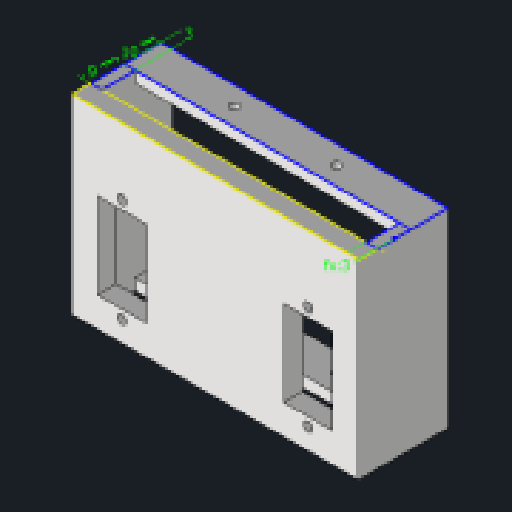
# Autodesk Inventor part: Test Frame
Saved by Autodesk Inventor 2023.2 (Build 272271030, 271C)
## iProperties
Created: 2023-10-24
Part Number: Test Frame
Material: Generic
Document SubType Name: Modeling
Designer: robpl
Density: 1 g/cm^3
Appearance: Default
Author: robpl
## iProperties of the stored document Test Frame_3DPrint.ipt
Created: 2023-10-25
Part Number: Test Frame_3DPrint
Material: Generic
Document SubType Name: Modeling
Designer: robpl
Density: 1 g/cm^3
Appearance: Default
Author: robpl
Autodesk Inventor part; units mm, degrees
ref_plane "YZ Plane" through (0, 0, 0) normal (1, 0, 0) x (0, 1, 0)
ref_plane "XZ Plane" through (0, 0, 0) normal (0, 1, 0) x (-1, 0, 0)
ref_plane "XY Plane" through (0, 0, 0) normal (0, 0, 1) x (1, 0, 0)
sketch "Sketch1" plane through (0, 0, 0) normal (0, 0, 1) x (1, 0, 0)
  line L0 (0, 0) -> (-77, 0)
  line L1 (-77, 0) -> (-77, -51.3)
  line L2 (-77, -51.3) -> (0, -51.3)
  line L3 (0, -51.3) -> (0, 0)
  line L4 (-7, -20.3) -> (-20, -20.3)
  line L5 (-20, -20.3) -> (-20, -43.3)
  line L6 (-20, -43.3) -> (-7, -43.3)
  line L7 (-7, -43.3) -> (-7, -20.3)
  line L8 (-57, -20.3) -> (-70, -20.3)
  line L9 (-70, -20.3) -> (-70, -43.3)
  line L10 (-70, -43.3) -> (-57, -43.3)
  line L11 (-57, -43.3) -> (-57, -20.3)
  point P0 (-7, -31.8)
  point P1 (0, -25.65)
  point P2 (-13.5, -20.3)
  point P3 (-63.5, -20.3)
  dimension "d1" = 51.3
  dimension "d4" = 23
  dimension "d5" = 13
  dimension "d7" = 7
  dimension "d18" = 50
  dimension "d19" = 7
  dimension "d20" = 8
  constraints: 24 end point, 6 parallel, 4 midpoint, 3 horizontal, 3 perpendicular, 2 equal length, 1 horizontal alignment
  measures "d1" distance of L1.end L0.end
  measures "d4" distance of L6.end L4.start
  measures "d5" distance of L4.start L4.end
  measures "d7" distance between parallel lines of L3 L7
  measures "d18" distance of point (-13.5, -20.3) point (-63.5, -20.3)
  measures "d19" distance between parallel lines of L1 L9
  measures "d20" distance between parallel lines of L2 L6
extrude "Extrusion1" add sketch "Sketch1" along normal blind 5
sketch "Sketch3" plane through (0, 0, 5) normal (0, 0, 1) x (1, 0, 0)
  line L0 (-77, 0) -> (-77, -51.3) projected
  line L1 (-77, -51.3) -> (0, -51.3) projected
  line L2 (0, -51.3) -> (0, 0) projected
  line L3 (0, 0) -> (-77, 0) projected
  line L4 (-7, -20.3) -> (-7, -43.3) projected
  line L5 (-7, -43.3) -> (-20, -43.3) projected
  line L6 (-20, -43.3) -> (-20, -20.3) projected
  line L7 (-20, -20.3) -> (-7, -20.3) projected
  line L8 (-20, -20.3) -> (-7, -20.3) projected
  line L9 (-70, -20.3) -> (-57, -20.3) projected
  point P0 (-13.5, -17.9)
  point P1 (-13.5, -45.7)
  point P2 (-13.5, -20.3)
  point P3 (-13.5, -20.3)
  point P4 (-13.5, -43.3)
  point P5 (-63.5, -17.9)
  point P6 (-63.5, -45.7)
  point P7 (-63.5, -20.3)
  point P8 (-63.5, -20.3)
  dimension "d8" = 27.8
  dimension "d9" = 2.4
  dimension "d10" = 2.4
  constraints: 5 midpoint, 4 vertical alignment, 2 horizontal alignment
  measures "d8" distance of point (-13.5, -17.9) point (-13.5, -45.7)
  measures "d9" distance from line of L7 point (-13.5, -17.9)
  measures "d10" distance of point (-13.5, -45.7) point (-13.5, -43.3)
hole "Hole1" at (-13.5, -17.9, 5) at (-13.5, -45.7, 5) at (-63.5, -45.7, 5) at (-63.5, -17.9, 5) direction (0, 0, -1) diameter 2.5 end through all
sketch "Sketch4" plane through (-77, 0, 0) normal (0, 1, 0) x (1, 0, 0)
  line L0 (77, 0) -> (0, 0) projected
  line L1 (0, 0) -> (0, -5) projected
  line L2 (77, -5) -> (0, -5) projected
  line L3 (77, 0) -> (77, -5) projected
  line L4 (77, 20) -> (0, 20)
  line L5 (0, 20) -> (0, 8)
  line L6 (0, 8) -> (77, 8)
  line L7 (77, 8) -> (77, 20)
  line L8 (0, 0) -> (77, 0) projected
  line L9 (77, 8) -> (57, 8)
  line L10 (57, 8) -> (57, 0)
  line L11 (57, 0) -> (77, 0)
  line L12 (77, 0) -> (77, 8)
  line L13 (0, 0) -> (20, 0)
  line L14 (20, 0) -> (20, 8)
  line L15 (20, 8) -> (0, 8)
  line L16 (0, 8) -> (0, 0)
  circle A0 centre (27.25, 13.95) radius 3.25
  point P0 (77, 4)
  point P1 (57, 8)
  dimension "d21" = 12
  dimension "d22" = 8
  dimension "d23" = 20
  dimension "d24" = 20
  dimension "d41" = 5.95
  constraints: 24 end point, 6 parallel, 3 horizontal, 3 perpendicular, 2 point on line, 2 vertical alignment, 1 centre point, 1 midpoint, 2 other
  measures "d21" distance of L4.end L5.end
  measures "d22" distance between parallel lines of L0 L6
  measures "d23" distance between parallel lines of L16 L14
  measures "d24" distance from line of point (77, 4) L10
  measures "d41" distance from line of L6 A0.centre
extrude "Extrusion2" add sketch "Sketch4" against normal blind 3 contours L0 L10 L6 L12 | L6 L5 L4 L7 | L0 L16 L6 L14 | A0
extrude "Extrusion3" add sketch "Sketch4" along normal blind 3 from surface at -51.3 contours L0 L10 L6 L12 | L6 L5 L4 L7 | L0 L16 L6 L14 | A0
sketch "Sketch5" plane through (0, 0, 0) normal (0, 0, -1) x (-1, 0, 0)
  line L0 (0, 0) -> (77, 0) projected
  line L1 (0, 0) -> (0, -3) projected
  line L2 (77, -3) -> (0, -3) projected
  line L3 (77, 0) -> (77, -3) projected
  line L4 (20, 0) -> (20, -3) projected
  line L5 (57, 0) -> (57, -3) projected
  line L6 (0, -48.3) -> (77, -48.3) projected
  line L7 (20, -3) -> (0, -3)
  line L8 (0, -3) -> (0, -48.3)
  line L9 (0, -48.3) -> (20, -48.3)
  line L10 (20, -48.3) -> (20, -3)
  line L11 (20, -3) -> (57, -3) projected
  line L12 (57, -3) -> (77, -3)
  line L13 (77, -3) -> (77, -48.3)
  line L14 (77, -48.3) -> (57, -48.3)
  line L15 (57, -48.3) -> (57, -3)
  line L16 (0, -3) -> (3, -3)
  line L17 (3, -3) -> (3, -48.3)
  line L18 (3, -48.3) -> (0, -48.3)
  line L19 (0, -48.3) -> (0, -3)
  line L20 (77, -3) -> (74, -3)
  line L21 (74, -3) -> (74, -48.3)
  line L22 (74, -48.3) -> (77, -48.3)
  line L23 (77, -48.3) -> (77, -3)
  point P0 (0, -3)
  point P1 (20, -48.3)
  point P2 (3, -48.3)
  dimension "d42" = 3
  dimension "d43" = 3
  constraints: 32 end point, 8 parallel, 4 horizontal, 4 perpendicular, 2 point on line
  measures "d42" distance between parallel lines of L19 L17
  measures "d43" distance between parallel lines of L13 L21
extrude "Extrusion4" add sketch "Sketch5" along normal up to surface (20 mm away) contours L2 L17 L6 L8 | L13 L6 L21 L2
sketch "Sketch6" plane through (-77, 0, 5) normal (0, 1, 0) x (1, 0, 0)
  line L0 (20, 5) -> (20, 13) projected
  line L1 (20, 13) -> (57, 13) projected
  line L2 (57, 13) -> (57, 5) projected
  line L3 (57, 5) -> (20, 5) projected
  line L4 (0, 25) -> (0, 0) projected
  line L5 (77, 0) -> (0, 0) projected
  line L6 (77, 25) -> (77, 0) projected
  line L7 (77, 25) -> (0, 25) projected
  point P0 (77, 5)
  point P1 (49.75, 18.95)
  point P2 (27.25, 18.95)
  dimension "d31" = 27.25
  dimension "d32" = 27.25
  dimension "d33" = 6.05
  constraints: 1 horizontal alignment
  measures "d31" distance from line of L6 point (49.75, 18.95)
  measures "d32" distance from line of L4 point (27.25, 18.95)
  measures "d33" distance from line of L7 point (49.75, 18.95)
hole "Hole2" at (-27.25, 0, -13.95) at (-49.75, 0, -13.95) direction (0, -1, 0) diameter 6.5 end through all
equation "\"d19\" = d7"
equation "\"d10\" = d9"
equation "\"d23\" = d24"
equation "\"d43\" = d42"
equation "\"d32\" = d31"
body "Solid1"
